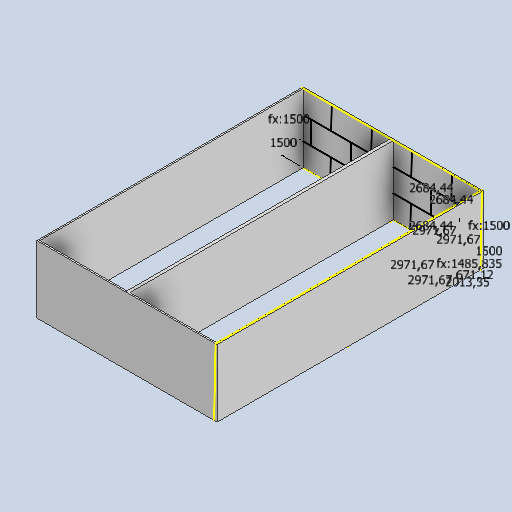
# Autodesk Inventor part: GBK overall model
Saved by Autodesk Inventor 2026 (Build 300175000, 175)
## iProperties
Created: 2026-05-17
Part Number: GBK overall model
Material: Типовые
Document SubType Name: Modeling
Designer: pokla
Density: 1 g/cm^3
Appearance: По умолчанию
Author: pokla
Autodesk Inventor part; units mm, degrees
ref_plane "YZ Plane" through (0, 0, 0) normal (1, 0, 0) x (0, 1, 0)
ref_plane "XZ Plane" through (0, 0, 0) normal (0, 1, 0) x (-1, 0, 0)
ref_plane "XY Plane" through (0, 0, 0) normal (0, 0, 1) x (1, 0, 0)
sketch "Эскиз1" plane through (0, 0, 0) normal (0, 1, 0) x (-1, 0, 0)
  line L0 (6040, 8925) -> (-6040, 8925)
  line L1 (-6040, 8925) -> (-6040, -8925)
  line L2 (-6040, -8925) -> (6040, -8925)
  line L3 (6040, -8925) -> (6040, 8925)
  line L4 (-6040, 8925) -> (6040, -8925) construction
  line L5 (-5840, 8725) -> (-5840, -8725)
  line L6 (5840, -8725) -> (5840, 8725)
  line L7 (200, 8725) -> (200, -8725)
  line L8 (-200, 8725) -> (-200, -8725)
  line L9 (5840, 8725) -> (200, 8725)
  line L10 (-200, 8725) -> (-5840, 8725)
  line L11 (-5840, -8725) -> (-200, -8725)
  line L12 (200, -8725) -> (5840, -8725)
  point P0 (0, 0)
  point P1 (0, 0)
  dimension "d0" = 12080
  dimension "d1" = 17850
  dimension "d5" = 200
  dimension "d6" = 400
  dimension "d7" = 200
  dimension "d16" = 200
  dimension "d17" = 200
  dimension "d18" = 200
  constraints: 26 end point, 7 parallel, 7 perpendicular, 2 collinear, 1 coincident, 1 horizontal, 1 midpoint
  measures "d0" distance between parallel lines of L1 L3
  measures "d1" distance between parallel lines of L2 L0
  measures "d5" distance between parallel lines of L3 L6
  measures "d6" distance between parallel lines of L8 L7
  measures "d7" distance from line of point (0, 0) L7
  measures "d16" distance between parallel lines of L0 L9
  measures "d17" distance between parallel lines of L2 L12
  measures "d18" distance between parallel lines of L1 L5
extrude "Выдавливание4" add sketch "Эскиз1" along normal blind 4500
sketch "Эскиз3" plane through (0, 4500, 0) normal (0, 1, 0) x (1, 0, 0)
  line L0 (6040, -8925) -> (6040, 8925) projected
  line L1 (6040, 8925) -> (-6040, 8925) projected
  line L2 (-6040, 8925) -> (-6040, -8925) projected
  line L3 (-6040, -8925) -> (6040, -8925) projected
  line L4 (200, -8725) -> (200, 8725) projected
  line L5 (200, 8725) -> (5840, 8725) projected
  line L6 (5840, 8725) -> (5840, -8725) projected
  line L7 (5840, -8725) -> (200, -8725) projected
  line L8 (-5840, 8725) -> (-200, 8725) projected
  line L9 (-200, 8725) -> (-200, -8725) projected
  line L10 (-200, -8725) -> (-5840, -8725) projected
  line L11 (-5840, -8725) -> (-5840, 8725) projected
  line L12 (-5940, 8825) -> (-100, 8825)
  line L13 (-100, 8825) -> (-100, -8825)
  line L14 (-100, -8825) -> (-5940, -8825)
  line L15 (-5940, -8825) -> (-5940, 8825)
  line L16 (100, 8825) -> (100, -8825)
  line L17 (100, -8825) -> (5940, -8825)
  line L18 (5940, -8825) -> (5940, 8825)
  line L19 (5940, 8825) -> (100, 8825)
  point P0 (0, 0)
  dimension "d25" = 100
  dimension "d26" = 100
  constraints: 16 end point, 6 other
  measures "d25" distance between parallel lines of L11 L15
  measures "d26" distance between parallel lines of L4 L16
loft "Лофт1" cut profiles "Эскиз3", "Эскиз1" contours L4 L5 L6 L7 | L19 L18 L17 L16 / L10 L8 L11 L5
loft "Лофт2" cut profiles "Эскиз3", "Эскиз1" contours L8 L9 L10 L11 | L12 L13 L14 L15 / L12 L7 L9 L6
sketch "Эскиз4" plane through (5840, 0, -8725) normal (-0.9998, 0.0222, 0) x (0, 0, 1)
  line L0 (17650, 4.4433) -> (-200, 4.4433) projected
  line L1 (-200, 4.4433) -> (-200, 4503.3326) projected
  line L2 (17650, 4503.3326) -> (-200, 4503.3326) projected
  line L3 (17650, 4.4433) -> (17650, 4503.3326) projected
  line L4 (-200, 1504.4433) -> (17650, 1504.4433)
  line L5 (-200, 3004.4433) -> (17650, 3004.4433)
  line L6 (2771.67, 3004.4433) -> (2771.67, 1504.4433)
  line L7 (1285.835, 1504.4433) -> (1285.835, 4.4433)
  line L8 (5743.34, 3004.4433) -> (5743.34, 1504.4433)
  line L9 (8715.01, 3004.4433) -> (8715.01, 1504.4433)
  line L10 (11686.68, 3004.4433) -> (11686.68, 1504.4433)
  line L11 (14658.35, 3004.4433) -> (14658.35, 1504.4433)
  line L12 (4257.505, 1504.4433) -> (4257.505, 4.4433)
  line L13 (7229.175, 1504.4433) -> (7229.175, 4.4433)
  line L14 (10200.845, 1504.4433) -> (10200.845, 4.4433)
  line L15 (13172.515, 1504.4433) -> (13172.515, 4.4433)
  line L16 (16144.185, 1504.4433) -> (16144.185, 4.4433)
  line L17 (1285.835, 3004.4433) -> (1285.835, 4503.3326)
  line L18 (17650, 4503.3326) -> (-200, 4503.3326) projected
  line L19 (4257.505, 3004.4433) -> (4257.505, 4503.3326)
  line L20 (7229.175, 3004.4433) -> (7229.175, 4503.3326)
  line L21 (10200.845, 3004.4433) -> (10200.845, 4503.3326)
  line L22 (13172.515, 3004.4433) -> (13172.515, 4503.3326)
  line L23 (16144.185, 3004.4433) -> (16144.185, 4503.3326)
  point P0 (8725, -129.7457)
  dimension "d38" = 1500
  dimension "d40" = 1500
  dimension "d41" = 2971.67
  dimension "d42" = 1485.835
  dimension "d45" = 2971.67
  dimension "d52" = 2971.67
  dimension "d59" = 2971.67
  constraints: 38 end point, 10 point on line, 5 perpendicular, 3 horizontal, 1 collinear, 42 other
  measures "d38" distance between parallel lines of L0 L4
  measures "d40" distance between parallel lines of L4 L5
  measures "d41" distance between parallel lines of L1 L6
  measures "d42" distance between parallel lines of L1 L7
  measures "d45" distance of L6.start L8.start
  measures "d52" distance of L7.start L12.start
  measures "d59" distance of L17.start L19.start
sketch "Эскиз5" plane through (200, 0, -8725) normal (0, 0.0222, 0.9998) x (1, 0, 0)
  line L0 (5840, 4.4433) -> (-6240, 4.4433) projected
  line L1 (-6240, 4.4433) -> (-6240, 4503.3326) projected
  line L2 (5840, 4503.3326) -> (-6240, 4503.3326) projected
  line L3 (5840, 4.4433) -> (5840, 4503.3326) projected
  line L4 (-6240, 1504.4433) -> (5840, 1504.4433)
  line L5 (-6240, 3004.4433) -> (5840, 3004.4433)
  line L6 (3826.65, 1504.4433) -> (3826.65, 4.4433)
  line L7 (5168.88, 3004.4433) -> (5168.88, 1504.4433)
  line L8 (3826.65, 3004.4433) -> (3826.65, 4503.3326)
  line L9 (1142.21, 1504.4433) -> (1142.21, 4.4433)
  line L10 (-1542.23, 1504.4433) -> (-1542.23, 4.4433)
  line L11 (-4226.67, 1504.4433) -> (-4226.67, 4.4433)
  line L12 (1142.21, 3004.4433) -> (1142.21, 4503.3326)
  line L13 (-1542.23, 3004.4433) -> (-1542.23, 4503.3326)
  line L14 (-4226.67, 3004.4433) -> (-4226.67, 4503.3326)
  line L15 (2484.44, 3004.4433) -> (2484.44, 1504.4433)
  line L16 (-200, 3004.4433) -> (-200, 1504.4433)
  line L17 (-2884.44, 3004.4433) -> (-2884.44, 1504.4433)
  line L18 (-5568.88, 3004.4433) -> (-5568.88, 1504.4433)
  point P0 (-200, -193.841)
  dimension "d64" = 1500
  dimension "d65" = 1500
  dimension "d66" = 2013.35
  dimension "d89" = 671.12
  dimension "d92" = 2684.44
  dimension "d99" = 2684.44
  dimension "d106" = 2684.44
  constraints: 30 end point, 10 point on line, 5 perpendicular, 3 horizontal, 1 collinear, 30 other
  measures "d64" distance between parallel lines of L0 L4
  measures "d65" distance between parallel lines of L4 L5
  measures "d66" distance between parallel lines of L3 L6
  measures "d89" distance between parallel lines of L7 L3
  measures "d92" distance of L6.start L9.start
  measures "d99" distance of L8.start L12.start
  measures "d106" distance of L7.start L15.start
equation "\"d40\" = d38"
equation "\"d42\" = 0.5 * d41"
equation "\"d65\" = d64"
